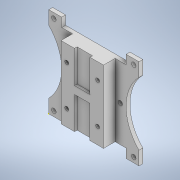
# Autodesk Inventor part: body
Saved by Autodesk Inventor 2022.2 (Build 262287010, 287A)
## iProperties
Created: 2022-02-20
Part Number: body
Material: Generic
Document SubType Name: Modeling
Designer: Nakai
Density: 1 g/cm^3
Appearance: Default
Author: Nakai
Autodesk Inventor part; units mm, degrees
ref_plane "YZ Plane" through (0, 0, 0) normal (1, 0, 0) x (0, 1, 0)
ref_plane "XZ Plane" through (0, 0, 0) normal (0, 1, 0) x (-1, 0, 0)
ref_plane "XY Plane" through (0, 0, 0) normal (0, 0, 1) x (1, 0, 0)
sketch "Sketch1" plane through (0, 0, 0) normal (0, 0, 1) x (1, 0, 0)
  line L0 (0, 0) -> (70, 0)
  line L1 (70, 0) -> (70, 70)
  line L2 (70, 70) -> (0, 70)
  line L3 (0, 70) -> (0, 0)
  dimension "d0" = 70
  dimension "d1" = 70
  constraints: 8 end point, 2 parallel, 1 horizontal, 1 perpendicular
  measures "d0" distance of L2.end L1.end
  measures "d1" distance of L1.end L0.end
extrude "Extrusion1" add sketch "Sketch1" along normal blind 3
sketch "Esboço3" plane through (0, 0, 3) normal (0, 0, 1) x (1, 0, 0)
  line L0 (70, 70) -> (0, 70) projected
  line L1 (70, 0) -> (70, 70) projected
  line L2 (0, 70) -> (0, 0) projected
  line L3 (41, 63) -> (29, 63)
  line L4 (29, 63) -> (29, 38)
  line L5 (29, 38) -> (41, 38)
  line L6 (41, 38) -> (41, 63)
  line L7 (41, 7) -> (29, 7)
  line L8 (29, 7) -> (29, 32)
  line L9 (29, 32) -> (41, 32)
  line L10 (41, 32) -> (41, 7)
  line L11 (0, 0) -> (70, 0) projected
  circle A0 centre (23, 19.5) radius 1.5
  circle A1 centre (23, 19.5) radius 4.5
  circle A2 centre (47, 19.5) radius 1.5
  circle A3 centre (47, 19.5) radius 4.5
  circle A4 centre (23, 50.5) radius 4.5
  circle A5 centre (23, 50.5) radius 1.5
  circle A6 centre (47, 50.5) radius 1.5
  circle A7 centre (47, 50.5) radius 4.5
  line L12 (18.5, 7) -> (51.5, 7)
  line L13 (51.5, 7) -> (51.5, 63)
  line L14 (51.5, 63) -> (18.5, 63)
  line L15 (18.5, 63) -> (18.5, 7)
  point P0 (35, 70)
  point P1 (35, 63)
  point P2 (35, 7)
  point P3 (29, 50.5)
  point P4 (35, 32)
  point P5 (18.5, 50.5)
  point P6 (18.5, 19.5)
  point P7 (51.5, 19.5)
  point P8 (51.5, 50.5)
  dimension "d10" = 70
  dimension "d11" = 12
  dimension "d12" = 25
  dimension "d13" = 7
  dimension "d14" = 35
  dimension "d15" = 12
  dimension "d16" = 25
  dimension "d17" = 7
  dimension "d18" = 35
  dimension "d21" = 3
  dimension "d22" = 12.5
  dimension "d24" = 9
  dimension "d25" = 6
  dimension "d26" = 3
  dimension "d27" = 9
  dimension "d28" = 6
  dimension "d29" = 12.5
  dimension "d30" = 9
  dimension "d31" = 6
  dimension "d32" = 3
  dimension "d33" = 12.5
  dimension "d34" = 3
  dimension "d35" = 9
  dimension "d36" = 12.5
  dimension "d37" = 6
  dimension "d40" = 56
  dimension "d41" = 16.5
  dimension "d42" = 16.5
  constraints: 24 end point, 8 centre point, 6 parallel, 5 midpoint, 4 coincident, 3 horizontal, 3 perpendicular
  measures "d10" distance between parallel lines of L2 L1
  measures "d11" distance of L5.end L4.end
  measures "d12" distance of L4.end L3.end
  measures "d13" distance from line of point (35, 70) L3
  measures "d14" distance from line of point (35, 63) L1
  measures "d15" distance of L8.end L9.end
  measures "d16" distance of L7.end L8.end
  measures "d17" distance between parallel lines of L11 L7
  measures "d18" distance from line of L1 point (35, 7)
  measures "d21" diameter of A0
  measures "d22" distance from line of L9 A0.centre
  measures "d24" diameter of A1
  measures "d25" distance from line of L8 A0.centre
  measures "d26" diameter of A2
  measures "d27" diameter of A3
  measures "d28" distance from line of A2.centre L10
  measures "d29" distance from line of L9 A2.centre
  measures "d30" diameter of A4
  measures "d31" distance of point (29, 50.5) A4.centre
  measures "d32" diameter of A5
  measures "d33" vertical distance of A4.centre L4.end
  measures "d34" diameter of A6
  measures "d35" diameter of A7
  measures "d36" distance from line of L5 A6.centre
  measures "d37" distance from line of L6 A6.centre
  measures "d40" distance between parallel lines of L14 L12
  measures "d41" distance from line of L15 point (35, 32)
  measures "d42" distance from line of L13 point (35, 32)
extrude "Extrusão4" add sketch "Esboço3" along normal blind 9 contours L6 L5 L4 L3 | A4 | A1 | A3 | A7 | L14 L13 L12 L10 L9 L8 L15 L4 L5 L6 | L7 L8 L9 L10
sketch "Esboço4" plane through (0, 0, 12) normal (0, 0, 1) x (1, 0, 0)
  line L0 (70, 70) -> (0, 70)
  line L1 (70, 0) -> (70, 70)
  line L2 (0, 70) -> (0, 0)
  line L3 (41, 63) -> (29, 63)
  line L4 (29, 63) -> (29, 38)
  line L5 (29, 38) -> (41, 38)
  line L6 (41, 38) -> (41, 63)
  line L7 (41, 7) -> (29, 7)
  line L8 (29, 7) -> (29, 32)
  line L9 (29, 32) -> (41, 32)
  line L10 (41, 32) -> (41, 7)
  line L11 (0, 0) -> (70, 0)
  circle A0 centre (23, 19.5) radius 1.5
  circle A1 centre (23, 19.5) radius 4.5
  circle A2 centre (47, 19.5) radius 1.5
  circle A3 centre (47, 19.5) radius 4.5
  circle A4 centre (23, 50.5) radius 4.5
  circle A5 centre (23, 50.5) radius 1.5
  circle A6 centre (47, 50.5) radius 1.5
  circle A7 centre (47, 50.5) radius 4.5
  line L12 (18.5, 7) -> (51.5, 7)
  line L13 (51.5, 7) -> (51.5, 63)
  line L14 (51.5, 63) -> (18.5, 63)
  line L15 (18.5, 63) -> (18.5, 7)
  point P0 (35, 70)
  point P1 (35, 63)
  point P2 (35, 7)
  point P3 (29, 50.5)
  point P4 (35, 32)
  point P5 (18.5, 50.5)
  point P6 (18.5, 19.5)
  point P7 (51.5, 19.5)
  point P8 (51.5, 50.5)
  dimension "d43" = 70
  dimension "d44" = 12
  dimension "d45" = 25
  dimension "d46" = 7
  dimension "d47" = 35
  dimension "d48" = 12
  dimension "d49" = 25
  dimension "d50" = 7
  dimension "d51" = 35
  dimension "d52" = 3
  dimension "d53" = 12.5
  dimension "d54" = 9
  dimension "d55" = 6
  dimension "d56" = 3
  dimension "d57" = 9
  dimension "d58" = 6
  dimension "d59" = 12.5
  dimension "d60" = 9
  dimension "d61" = 6
  dimension "d62" = 3
  dimension "d63" = 12.5
  dimension "d64" = 3
  dimension "d65" = 9
  dimension "d66" = 12.5
  dimension "d67" = 6
  dimension "d68" = 56
  dimension "d69" = 16.5
  dimension "d70" = 16.5
  constraints: 32 end point, 8 centre point, 6 parallel, 5 midpoint, 4 coincident, 3 horizontal, 3 perpendicular
  measures "d43" distance between parallel lines of L2 L1
  measures "d44" distance of L5.end L4.end
  measures "d45" distance of L4.end L3.end
  measures "d46" distance from line of point (35, 70) L3
  measures "d47" distance from line of point (35, 63) L1
  measures "d48" distance of L8.end L9.end
  measures "d49" distance of L7.end L8.end
  measures "d50" distance between parallel lines of L11 L7
  measures "d51" distance from line of L1 point (35, 7)
  measures "d52" diameter of A0
  measures "d53" distance from line of L9 A0.centre
  measures "d54" diameter of A1
  measures "d55" distance from line of L8 A0.centre
  measures "d56" diameter of A2
  measures "d57" diameter of A3
  measures "d58" distance from line of A2.centre L10
  measures "d59" distance from line of L9 A2.centre
  measures "d60" diameter of A4
  measures "d61" distance of point (29, 50.5) A4.centre
  measures "d62" diameter of A5
  measures "d63" vertical distance of A4.centre L4.end
  measures "d64" diameter of A6
  measures "d65" diameter of A7
  measures "d66" distance from line of L5 A6.centre
  measures "d67" distance from line of L6 A6.centre
  measures "d68" distance between parallel lines of L14 L12
  measures "d69" distance from line of L15 point (35, 32)
  measures "d70" distance from line of L13 point (35, 32)
extrude "Extrusão5" cut sketch "Esboço4" against normal blind 2 contours L6 L5 L4 L3 | L7 L8 L9 L10
sketch "Esboço5" plane through (0, 0, 3) normal (0, 0, 1) x (1, 0, 0)
  line L0 (0, 0) -> (70, 0) projected
  line L1 (10, 0) -> (60, 0)
  line L2 (60, 0) -> (60, 7)
  line L3 (60, 7) -> (10, 7)
  line L4 (10, 7) -> (10, 0)
  line L5 (70, 70) -> (0, 70) projected
  line L6 (10, 70) -> (60, 70)
  line L7 (60, 70) -> (60, 63)
  line L8 (60, 63) -> (10, 63)
  line L9 (10, 63) -> (10, 70)
  point P0 (35, 0)
  point P1 (60, 3.5)
  point P2 (10, 66.5)
  point P3 (35, 70)
  dimension "d73" = 50
  dimension "d74" = 25
  dimension "d75" = 7
  dimension "d76" = 50
  dimension "d77" = 7
  dimension "d78" = 25
  constraints: 16 end point, 4 midpoint, 4 parallel, 2 horizontal, 2 perpendicular, 2 point on line
  measures "d73" distance of L3.end L2.end
  measures "d74" horizontal distance of point (35, 0) point (60, 3.5)
  measures "d75" distance of L1.end L2.end
  measures "d76" distance of L7.end L8.end
  measures "d77" distance of L6.end L7.end
  measures "d78" horizontal distance of point (10, 66.5) point (35, 70)
extrude "Extrusão6" cut sketch "Esboço5" against normal up to surface (3 mm away)
sketch "Esboço6" plane through (0, 0, 3) normal (0, 0, 1) x (1, 0, 0)
  circle A0 centre (-25, 35) radius 35
  line L0 (0, 70) -> (0, 0) projected
  line L1 (0, 0) -> (10, 0) projected
  circle A1 centre (95, 35) radius 35
  line L2 (70, 0) -> (70, 70) projected
  line L3 (60, 0) -> (70, 0) projected
  circle A2 centre (4, 66) radius 1.75
  circle A3 centre (66, 66) radius 1.75
  circle A4 centre (4, 4) radius 1.75
  circle A5 centre (66, 4) radius 1.75
  line L4 (10, 70) -> (0, 70) projected
  line L5 (70, 70) -> (60, 70) projected
  circle A6 centre (14.5, 35) radius 1.75
  line L6 (18.5, 63) -> (18.5, 7) projected
  circle A7 centre (55.5, 35) radius 1.75
  line L7 (51.5, 7) -> (51.5, 63) projected
  point P0 (0, 35)
  point P1 (65, 0)
  point P2 (70, 10.5051)
  point P3 (70, 59.4949)
  point P4 (0, 59.4949)
  point P5 (0, 10.5051)
  dimension "d81" = 70
  dimension "d82" = 25
  dimension "d83" = 35
  dimension "d84" = 70
  dimension "d85" = 25
  dimension "d86" = 35
  dimension "d89" = 3.5
  dimension "d90" = 3.5
  dimension "d91" = 3.5
  dimension "d92" = 3.5
  dimension "d93" = 4
  dimension "d94" = 4
  dimension "d95" = 4
  dimension "d96" = 4
  dimension "d97" = 4
  dimension "d98" = 4
  dimension "d99" = 4
  dimension "d100" = 4
  dimension "d101" = 3.5
  dimension "d102" = 4
  dimension "d103" = 35
  dimension "d104" = 3.5
  dimension "d105" = 4
  dimension "d106" = 35
  constraints: 8 centre point, 2 midpoint
  measures "d81" diameter of A0
  measures "d82" distance of A0.centre point (0, 35)
  measures "d83" distance from line of L1 A0.centre
  measures "d84" diameter of A1
  measures "d85" distance from line of L2 A1.centre
  measures "d86" vertical distance of point (65, 0) A1.centre
  measures "d89" diameter of A2
  measures "d90" diameter of A3
  measures "d91" diameter of A4
  measures "d92" diameter of A5
  measures "d93" distance from line of L4 A2.centre
  measures "d94" distance from line of L0 A2.centre
  measures "d95" distance from line of L1 A4.centre
  measures "d96" distance from line of L0 A4.centre
  measures "d97" distance from line of L2 A5.centre
  measures "d98" distance from line of L3 A5.centre
  measures "d99" distance from line of L5 A3.centre
  measures "d100" distance from line of L2 A3.centre
  measures "d101" diameter of A6
  measures "d102" distance from line of L6 A6.centre
  measures "d103" distance from line of L1 A6.centre
  measures "d104" diameter of A7
  measures "d105" distance from line of A7.centre L7
  measures "d106" distance from line of L3 A7.centre
extrude "Extrusão7" cut sketch "Esboço6" against normal up to surface (3 mm away) contours A0 L0 | L2 A1 | A2 | A3 | A4 | A5 | A6 | A7 picked at (1.4165, 28.5928) picked at (66.7381, 33.7107)
sketch "Esboço7" plane through (0, 0, 3) normal (0, 0, 1) x (1, 0, 0)
  point P0 (0, 0)
equation "\"d13\" = d17"
equation "\"d14\" = 0.5 * d10"
equation "\"d18\" = d14"
equation "\"d30\" = d24"
equation "\"d31\" = d25"
equation "\"d32\" = d21"
equation "\"d33\" = d22"
equation "\"d34\" = d21"
equation "\"d35\" = d27"
equation "\"d36\" = d29"
equation "\"d37\" = d28"
equation "\"d46\" = d50"
equation "\"d47\" = 0.5 * d43"
equation "\"d51\" = d47"
equation "\"d60\" = d54"
equation "\"d61\" = d55"
equation "\"d62\" = d52"
equation "\"d63\" = d53"
equation "\"d64\" = d52"
equation "\"d65\" = d57"
equation "\"d66\" = d59"
equation "\"d67\" = d58"
equation "\"d74\" = 0.5 * d73"
equation "\"d78\" = 0.5 * d76"
equation "\"d90\" = d89"
body "Solid1"
